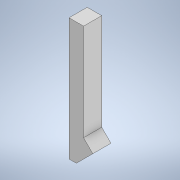
# Autodesk Inventor part: baseHook
Saved by Autodesk Inventor 2022 (Build 260153000, 153)
## iProperties
Created: 2022-08-24
Part Number: baseHook
Material: Generic
Document SubType Name: Modeling
Designer: sgioj
Density: 1 g/cm^3
Appearance: Default
Author: sgioj
Autodesk Inventor part; units mm, degrees
ref_plane "YZ Plane" through (0, 0, 0) normal (1, 0, 0) x (0, 1, 0)
ref_plane "XZ Plane" through (0, 0, 0) normal (0, 1, 0) x (-1, 0, 0)
ref_plane "XY Plane" through (0, 0, 0) normal (0, 0, 1) x (1, 0, 0)
sketch "Sketch1" plane through (0, 0, 0) normal (0, 0, 1) x (1, 0, 0)
  line L0 (2, -10.4654) -> (4.6978, -10.4654) construction
  line L1 (0, 0) -> (50, 0)
  line L2 (50, 0) -> (50, -50)
  line L3 (50, -50) -> (0, -50)
  line L4 (0, -50) -> (0, 0)
  line L5 (2.4, -2.4) -> (47.6, -2.4)
  line L6 (47.6, -2.4) -> (47.6, -47.6)
  line L7 (47.6, -47.6) -> (2.4, -47.6)
  line L8 (2.4, -47.6) -> (2.4, -2.4)
  line L9 (2.4, -2.4) -> (47.6, -47.6) construction
  line L10 (47.6, -2.4) -> (2.4, -47.6) construction
  circle A0 centre (25, -25) radius 19.375
  circle A1 centre (25, -25) radius 14.5
  circle A2 centre (25, -25) radius 4.175
  circle A3 centre (31.6798, -18.3202) radius 2.65
  circle A4 centre (25, -15.5534) radius 2.65
  circle A5 centre (18.3202, -18.3202) radius 2.65
  circle A6 centre (15.5534, -25) radius 2.65
  circle A7 centre (18.3202, -31.6798) radius 2.65
  circle A8 centre (25, -34.4466) radius 2.65
  circle A9 centre (31.6798, -31.6798) radius 2.65
  circle A10 centre (34.4466, -25) radius 2.65
  line L11 (50, -25) -> (-10.9328, -25) construction
  line L12 (33.5536, -16.4464) -> (35.253, -14.747)
  line L13 (33.5536, -33.5536) -> (35.253, -35.253)
  arc A11 (16.4464, -16.4464) -> (16.4475, -33.5547) centre (24.9923, -25) ccw
  line L14 (16.4464, -16.4464) -> (14.747, -14.747)
  line L15 (16.4475, -33.5547) -> (14.747, -35.253)
  line L16 (3.4, -3.4) -> (46.6, -3.4)
  line L17 (46.6, -3.4) -> (46.6, -46.6)
  line L18 (46.6, -46.6) -> (3.4, -46.6)
  line L19 (3.4, -46.6) -> (3.4, -3.4)
  line L20 (46.6, -46.6) -> (43.6, -46.6)
  line L21 (43.6, -46.6) -> (43.6, -43.6)
  line L22 (43.6, -43.6) -> (46.6, -43.6)
  line L23 (46.6, -43.6) -> (46.6, -46.6)
  line L24 (43.6, -43.6) -> (38.7002, -43.6)
  line L25 (38.7002, -43.6) -> (38.7002, -38.7002)
  line L26 (38.7002, -38.7002) -> (43.6, -38.7002)
  line L27 (43.6, -38.7002) -> (43.6, -43.6)
  line L28 (43.6, -38.7002) -> (46.6, -38.7002)
  line L29 (46.6, -38.7002) -> (46.6, -35.7002)
  line L30 (46.6, -35.7002) -> (43.6, -35.7002)
  line L31 (43.6, -35.7002) -> (43.6, -38.7002)
  line L32 (46.6, -35.7002) -> (42.8209, -35.7002)
  line L33 (42.8209, -35.7002) -> (42.8209, -32.6031)
  line L34 (42.8209, -32.6031) -> (46.6, -32.6031)
  line L35 (46.6, -32.6031) -> (46.6, -35.7002)
  line L36 (38.7002, -43.6) -> (35.7002, -43.6)
  line L37 (35.7002, -43.6) -> (35.7002, -46.6)
  line L38 (35.7002, -46.6) -> (38.7002, -46.6)
  line L39 (38.7002, -46.6) -> (38.7002, -43.6)
  line L40 (35.7002, -46.6) -> (32.3837, -46.6)
  line L41 (32.3837, -46.6) -> (32.3837, -42.9129)
  line L42 (32.3837, -42.9129) -> (35.7002, -42.9129)
  line L43 (35.7002, -42.9129) -> (35.7002, -46.6)
  line L44 (23.5, -43.2) -> (26.5, -43.2)
  line L45 (26.5, -43.2) -> (26.5, -50)
  line L46 (26.5, -50) -> (23.5, -50)
  line L47 (23.5, -50) -> (23.5, -43.2)
  line L48 (23.5, -43.2) -> (26.5, -50) construction
  line L49 (26.5, -43.2) -> (23.5, -50) construction
  circle A12 centre (7.9474, -7.9474) radius 4.5474
  circle A13 centre (42.0526, -7.9474) radius 4.5474
  line L50 (2.4, -47.6) -> (2.4, -50)
  line L51 (47.6, -47.6) -> (47.6, -50)
  line L52 (22.4071, -14.2334) -> (20.1941, -16.4464)
  line L53 (25, 8.5218) -> (25, -70.2) construction
  line L54 (18.3202, -8.8329) -> (18.3202, -33.5547) construction
  line L55 (18.3202, -14.5726) -> (20.1941, -16.4464)
  line L56 (18.3202, -14.5726) -> (20.5333, -12.3595)
  line L57 (22.4071, -14.2334) -> (20.5333, -12.3595)
  line L58 (18.3202, -14.5726) -> (19.593, -13.2998)
  line L59 (19.593, -13.2998) -> (20.8658, -14.5726)
  line L60 (20.8658, -14.5726) -> (19.593, -15.8454)
  line L61 (31.6798, -14.5726) -> (29.4667, -12.3595)
  line L62 (27.5929, -14.2334) -> (29.4667, -12.3595)
  line L63 (27.5929, -14.2334) -> (29.8059, -16.4464)
  line L64 (31.6798, -14.5726) -> (29.8059, -16.4464)
  line L65 (19.593, 0) -> (17.593, 0)
  line L66 (17.593, 0) -> (17.593, -16.837)
  line L67 (17.593, -16.837) -> (19.593, -16.837)
  line L68 (19.593, -16.837) -> (19.593, 0)
  line L69 (19.593, -15.8454) -> (18.6014, -16.837)
  point P0 (25, -46.6)
  point P1 (26.5, -44.3168)
  point P2 (26.5, -46.6)
  point P3 (42.0526, -3.4)
  point P4 (46.6, -7.9474)
  point P5 (3.4, -7.9474)
  point P6 (7.9474, -3.4)
  point P7 (26.5, -47.6)
  point P8 (23.5, -47.6)
  dimension "d12" = 5.3
  dimension "d5" = 50
  dimension "d6" = 50
  dimension "d7" = 45.2
  dimension "d8" = 45.2
  dimension "d9" = 38.75
  dimension "d10" = 29
  dimension "d11" = 8.35
  dimension "d13" = 360
  dimension "d14" = 2.4
  dimension "d15" = 2.4
  dimension "d16" = 1
  dimension "d17" = 1
  dimension "d18" = 1
  dimension "d19" = 3
  dimension "d20" = 3
  dimension "d21" = 3
  dimension "d22" = 3
  dimension "d23" = 3
  dimension "d24" = 3
  dimension "d25" = 3
  dimension "d26" = 1.8
  dimension "d27" = 2
  constraints: 138 end point, 22 parallel, 16 perpendicular, 14 point on line, 13 horizontal, 11 centre point, 11 point on circle, 5 coincident, 5 midpoint, 4 symmetric about line, 2 tangent, 2 vertical, 39 other
  measures "d5" distance of L2.end L3.end
  measures "d6" distance of L1.end L2.end
  measures "d7" distance of L6.end L7.end
  measures "d8" distance of L5.end L6.end
  measures "d9" diameter of A0
  measures "d10" diameter of A1
  measures "d11" diameter of A2
  measures "d14" distance between parallel lines of L4 L8
  measures "d15" distance between parallel lines of L1 L5
  measures "d16" distance between parallel lines of L16 L5
  measures "d17" distance between parallel lines of L8 L19
  measures "d18" distance between parallel lines of L18 L7
  measures "d19" distance of L21.end L22.end
  measures "d20" distance of L20.end L21.end
  measures "d21" distance of L30.end L29.end
  measures "d22" distance of L29.end L28.end
  measures "d23" distance of L38.end L37.end
  measures "d24" distance of L37.end L36.end
  measures "d25" distance of L45.end L46.end
  measures "d26" distance of L55.start L58.end
  measures "d27" distance of L67.end L66.end
extrude "Extrusion1" add sketch "Sketch1" along normal blind 2.5 contours L1 L68 L5 L66 | L5 L68 L16 L66 | L16 L68 A0 L66 | A0 L68 A1 L66 | A1 L68 L56 L55 L69 A5 L66 | A5 L69 L67 L66 | L68 L55 L56 | L59 L60 L68
body "Solid1"
